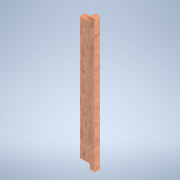
# Autodesk Inventor part: MagnetHolder
Saved by Autodesk Inventor 2022.2 (Build 262287000, 287)
## iProperties
Created: 2023-02-28
Part Number: MagnetHolder
Material: Wood (Oak)
Document SubType Name: Modeling
Designer: jaege
Density: 0.76 g/cm^3
Appearance: Red Oak - Natural Low Gloss
Author: jaege
Autodesk Inventor part; units mm, degrees
ref_plane "YZ Plane" through (0, 0, 0) normal (1, 0, 0) x (0, 1, 0)
ref_plane "XZ Plane" through (0, 0, 0) normal (0, 1, 0) x (-1, 0, 0)
ref_plane "XY Plane" through (0, 0, 0) normal (0, 0, 1) x (1, 0, 0)
sketch "Sketch1" plane through (0, 0, 0) normal (0, 0, 1) x (1, 0, 0)
  line L0 (0, 54) -> (-4, 54)
  line L1 (-4, 54) -> (-4, 50)
  line L2 (-4, -54) -> (0, -54)
  line L3 (0, -54) -> (0, 54)
  line L4 (-4, 50) -> (-12, 50)
  line L5 (-12, 50) -> (-12, -50)
  line L6 (-12, -50) -> (-4, -50)
  line L7 (-4, -50) -> (-4, 50) construction
  line L8 (-4, 50) -> (-4, -50) construction
  line L9 (-4, -50) -> (-4, -54)
  point P0 (0, 0)
  point P1 (-2, 54)
  point P2 (-2, -54)
  point P3 (-8, -50)
  point P4 (0, 0)
  dimension "d0" = 4
  dimension "d1" = 108
  dimension "d2" = 4
  dimension "d3" = 4
  dimension "d4" = 8
  constraints: 20 end point, 6 parallel, 4 midpoint, 4 perpendicular, 2 horizontal, 1 coincident
  measures "d0" distance of L0.start L0.end
  measures "d1" distance of L2.end L0.start
  measures "d2" distance from line of point (-2, 54) L4
  measures "d3" vertical distance of point (-2, -54) point (-8, -50)
  measures "d4" distance of L1.end L4.end
extrude "Extrusion1" add sketch "Sketch1" along normal blind 4
body "Solid1"
